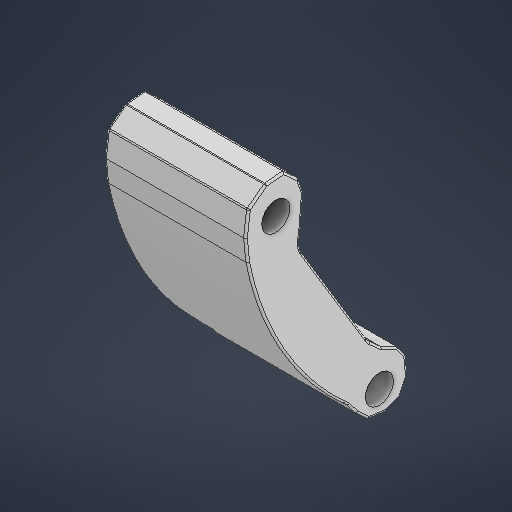
# Autodesk Inventor part: Lankarm_lång
Saved by Autodesk Inventor 2026 (Build 300175000, 175)
## iProperties
Created: 2025-04-29
Part Number: Lankarm_lång
Material: Generic
Document SubType Name: Modeling
Designer: elias
Density: 1 g/cm^3
Appearance: Default
Author: elias
Autodesk Inventor part; units mm, degrees
ref_plane "YZ Plane" through (0, 0, 0) normal (1, 0, 0) x (0, 1, 0)
ref_plane "XZ Plane" through (0, 0, 0) normal (0, 1, 0) x (-1, 0, 0)
ref_plane "XY Plane" through (0, 0, 0) normal (0, 0, 1) x (1, 0, 0)
sketch "Sketch1" plane through (0, 0, 0) normal (1, 0, 0) x (0, 1, 0)
  line L0 (2812.3869, 0) -> (2812.3869, -5171.1623) construction
  line L1 (2812.3869, -5171.1623) -> (0, -5171.1623) construction
  line L2 (0, -5171.1623) -> (0, 0) construction
  line L3 (0, 0) -> (2812.3869, 0) construction
  point P0 (0, 0)
  constraints: 2 end point, 2 other
sketch "Sketch3" plane through (0, 0, 0) normal (1, 0, 0) x (0, 1, 0)
  arc A0 (670.9217, -1192.002) -> (490.3182, -1294.4333) centre (735.6427, -1516.5486) ccw
  circle A1 centre (699.299, -1221.9874) radius 15
  circle A2 centre (485.0015, -1332.1305) radius 15
  line L0 (670.9217, -1192.002) -> (694.5217, -1189.6422)
  line L1 (694.5217, -1189.6422) -> (719.5378, -1192.8832)
  line L2 (719.5378, -1192.8832) -> (733.6455, -1211.4411)
  line L3 (733.6455, -1211.4411) -> (735.5916, -1230.9034)
  line L4 (735.5916, -1230.9034) -> (721.8585, -1246.2211)
  line L5 (721.8585, -1246.2211) -> (706.6308, -1251.2582)
  line L6 (706.6308, -1251.2582) -> (677.2013, -1248.7397)
  line L7 (677.2013, -1248.7397) -> (657.762, -1246.2211)
  line L8 (657.762, -1246.2211) -> (534.9682, -1320.4431)
  line L9 (534.9682, -1320.4431) -> (521.9986, -1334.9093)
  line L10 (521.9986, -1334.9093) -> (513.5108, -1351.8536)
  line L11 (513.5108, -1351.8536) -> (502.7761, -1360.014)
  line L12 (502.7761, -1360.014) -> (482.1715, -1362.0744)
  line L13 (482.1715, -1362.0744) -> (466.9183, -1354.4337)
  line L14 (466.9183, -1354.4337) -> (460.8027, -1339.4632)
  line L15 (460.8027, -1339.4632) -> (463.2669, -1320.4431)
  line L16 (463.2669, -1320.4431) -> (474.5449, -1307.8638)
  line L17 (474.5449, -1307.8638) -> (486.2652, -1298.954)
  line L18 (486.2652, -1298.954) -> (490.3182, -1294.4333)
  point P0 (0, 0)
  dimension "d9" = 30
  dimension "d10" = 30
  constraints: 38 end point, 6 parallel, 4 perpendicular, 3 centre point, 2 point on circle
  measures "d9" diameter of A1
  measures "d10" diameter of A2
extrude "Extrusion2" add sketch "Sketch3" along normal mid plane 150
fillet "Fillet1" radius 20 2 edges at (0, 657.762, -1246.2211) (0, 534.9682, -1320.4431)
fillet "Fillet2" radius 2 42 edges at (75, 572.3788, -1228.6872) (75, 488.2917, -1296.6937) (75, 480.405, -1303.4089) (75, 468.9059, -1314.1535) (75, 462.0348, -1329.9531) (75, 463.8605, -1346.9484) (75, 474.5449, -1358.254) (75, 492.4738, -1361.0442) (75, 508.1435, -1355.9338) (75, 517.7547, -1343.3815) (75, 527.4874, -1328.7871) (75, 535.1095, -1320.6136) (75, 594.6506, -1284.3684) (75, 670.948, -1247.9295) (75, 691.916, -1249.9989) (75, 714.2446, -1248.7397) (75, 728.725, -1238.5623) (75, 734.6185, -1221.1723) (75, 726.5916, -1202.1622) (75, 707.0298, -1191.2627) (75, 682.7217, -1190.8221) (-75, 572.3788, -1228.6872) (-75, 682.7217, -1190.8221) (-75, 707.0298, -1191.2627) (-75, 726.5916, -1202.1622) (-75, 734.6185, -1221.1723) (-75, 728.725, -1238.5623) (-75, 714.2446, -1248.7397) (-75, 691.916, -1249.9989) (-75, 670.948, -1247.9295) (-75, 594.6506, -1284.3684) (-75, 535.1095, -1320.6136) (-75, 527.4874, -1328.7871) (-75, 517.7547, -1343.3815) (-75, 508.1435, -1355.9338) (-75, 492.4738, -1361.0442) (-75, 474.5449, -1358.254) (-75, 463.8605, -1346.9484) (-75, 462.0348, -1329.9531) (-75, 468.9059, -1314.1535) (-75, 480.405, -1303.4089) (-75, 488.2917, -1296.6937)
fillet "Fillet3" radius 2 6 edges at (0, 719.5378, -1192.8832) (0, 733.6455, -1211.4411) (74.4142, 719.2197, -1193.4327) (-74.4142, 719.2197, -1193.4327) (74.4142, 733.079, -1211.6639) (-74.4142, 733.079, -1211.6639)
body "Solid2"
